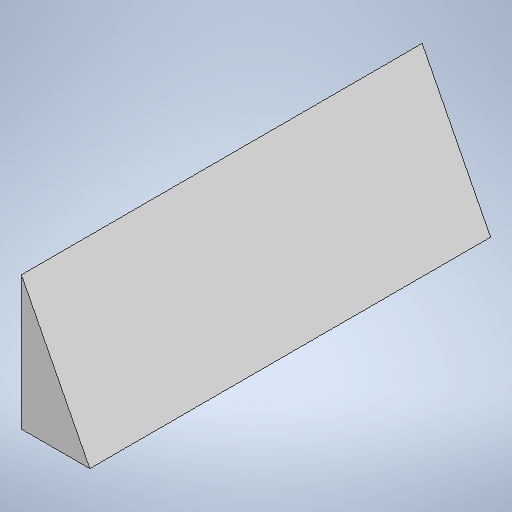
# Autodesk Inventor part: ABREBOTELLAS INDIVIDUAL FIDE1.0
Saved by Autodesk Inventor 2025.1 (Build 291241000, 241)
## iProperties
Created: 2024-11-02
Part Number: ABREBOTELLAS INDIVIDUAL FIDE1.0
Material: Genérico
Document SubType Name: Modeling
Designer: Octavio
Density: 1 g/cm^3
Appearance: Valor por defecto
Author: Octavio
Autodesk Inventor part; units mm, degrees
ref_plane "YZ Plane" through (0, 0, 0) normal (1, 0, 0) x (0, 1, 0)
ref_plane "XZ Plane" through (0, 0, 0) normal (0, 1, 0) x (-1, 0, 0)
ref_plane "XY Plane" through (0, 0, 0) normal (0, 0, 1) x (1, 0, 0)
sketch "Boceto1" plane through (0, 0, 0) normal (0, 0, 1) x (1, 0, 0)
  line L0 (0, 0) -> (1.281, 0)
  line L1 (1.281, 0) -> (0, 2.5)
  line L2 (0, 2.5) -> (0, 0)
  dimension "d0" = 1.281
  dimension "d1" = 2.5
  constraints: 6 end point, 1 horizontal, 1 perpendicular
  measures "d0" distance of L0.start L0.end
  measures "d1" distance of L1.end L0.start
extrude "Extrusión1" add sketch "Boceto1" along normal blind 7.5
